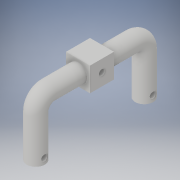
# Autodesk Inventor part: bogie (1)
Saved by Autodesk Inventor 2017 (Build 210142000, 142)
## iProperties
Created: 2017-10-30
Part Number: bogie (1)
Material: Generic
Document SubType Name: Modeling
Designer: 602199
Density: 1 g/cm^3
Appearance: Default
Author: 602199
Autodesk Inventor part; units mm, degrees
ref_plane "YZ Plane" through (0, 0, 0) normal (1, 0, 0) x (0, 1, 0)
ref_plane "XZ Plane" through (0, 0, 0) normal (0, 1, 0) x (-1, 0, 0)
ref_plane "XY Plane" through (0, 0, 0) normal (0, 0, 1) x (1, 0, 0)
sketch "Sketch1" plane through (0, 0, 0) normal (0, 1, 0) x (-1, 0, 0)
  circle A0 centre (0, 0) radius 19.05
  dimension "d0" = 38.1
  constraints: 1 centre point, 1 coincident
  measures "d0" diameter of A0
sketch "Sketch2" plane through (0, 0, 0) normal (1, 0, 0) x (0, 1, 0)
  line L0 (0, 0) -> (88.9, 0)
  arc A0 (114.8745, -25.9745) -> (88.9, 0) centre (88.9, -25.9745) ccw
  line L1 (114.8745, -25.9745) -> (114.8745, -203.7745)
  line L2 (0, -229.749) -> (88.9, -229.749)
  arc A1 (88.9, -229.749) -> (113.9345, -210.699) centre (88.9, -203.7745) ccw
  arc A2 (88.9, -229.749) -> (114.8745, -203.7745) centre (88.9, -203.7745) ccw
  dimension "d2" = 88.9
  constraints: 6 end point, 6 point on circle, 3 centre point, 1 coincident, 1 tangent, 1 vertical
  measures "d2" distance of L0.start L0.end
sweep "Sweep1" add profiles "Sketch1" path "Sketch2" path curves L0 A0 L1 A2 L2
sketch "Sketch3" plane through (0, 0, 0) normal (1, 0, 0) x (0, 1, 0)
  line L0 (95.8245, -25.9745) -> (133.9245, -25.9745) projected
  line L1 (133.9245, -25.9745) -> (133.9245, -203.7745)
  line L2 (133.9245, -25.9745) -> (133.9245, -203.7745) projected
  line L3 (133.9245, -114.8745) -> (95.8245, -114.8745)
  line L4 (95.8245, -25.9745) -> (95.8245, -203.7745) projected
  line L5 (89.4745, -89.4745) -> (140.2745, -89.4745)
  line L6 (140.2745, -89.4745) -> (140.2745, -140.2745)
  line L7 (140.2745, -140.2745) -> (89.4745, -140.2745)
  line L8 (89.4745, -140.2745) -> (89.4745, -89.4745)
  line L9 (89.4745, -89.4745) -> (140.2745, -140.2745) construction
  line L10 (140.2745, -89.4745) -> (89.4745, -140.2745) construction
  point P0 (0, 0)
  point P1 (114.8745, -114.8745)
  dimension "d8" = 50.8
  dimension "d9" = 50.8
  constraints: 16 end point, 5 midpoint, 2 parallel, 1 horizontal, 1 perpendicular, 1 point on line
  measures "d8" distance of L6.end L7.end
  measures "d9" distance of L5.end L6.end
extrude "Extrusion1" add sketch "Sketch3" along normal mid plane 50.8 contours L5 L1 L3 L4 | L4 L7 L8 L5 | L5 L6 L7 L1 | L3 L1 L7 L4
sketch "Sketch4" plane through (25.4, 0, 0) normal (1, 0, 0) x (0, 0, -1)
  line L0 (140.2745, 140.2745) -> (89.4745, 140.2745) construction
  line L1 (114.8745, 140.2745) -> (114.8745, 89.4745) construction
  line L2 (89.4745, 89.4745) -> (140.2745, 89.4745) construction
  line L3 (140.2745, 95.8245) -> (140.2745, 133.9245) construction
  line L4 (140.2745, 114.8745) -> (89.4745, 114.8745) construction
  line L5 (89.4745, 133.9245) -> (89.4745, 95.8245) construction
  circle A0 centre (114.8745, 114.8745) radius 6.35
  point P0 (0, 0)
  dimension "d23" = 12.7
  constraints: 5 midpoint, 4 end point, 1 centre point
  measures "d23" diameter of A0
extrude "Extrusion2" cut sketch "Sketch4" against normal through all
sketch "Sketch5" plane through (0, 0, 0) normal (1, 0, 0) x (0, 1, 0)
  line L0 (0, 0) -> (12.7, 0)
  line L1 (0, 0) -> (12.7, 0) construction
  line L2 (140.2745, -140.2745) -> (140.2745, -89.4745) projected
  line L3 (140.2745, -114.8745) -> (3.175, -114.8745)
  circle A0 centre (12.7, 0) radius 6.35
  circle A1 centre (12.7, -229.749) radius 6.35
  dimension "d16" = 12.7
  dimension "d21" = 12.7
  dimension "d22" = 12.7
  constraints: 6 end point, 3 horizontal, 2 centre point, 1 coincident, 1 collinear, 1 midpoint
  measures "d16" distance of L0.start L0.end
  measures "d21" diameter of A0
  measures "d22" diameter of A1
extrude "Extrusion3" cut sketch "Sketch5" along normal through all both and the other way through all
body "Solid1"
